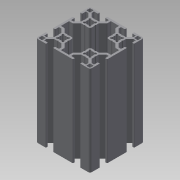
# Autodesk Inventor part: 30-6060
Saved by Autodesk Inventor 2013 (Build 170138000, 138)
## iProperties
Created: 2014-04-23
Part Number: 30-6060
Material: Generic
Document SubType Name: Modeling
Designer: Ross Bowman
Density: 1 g/cm^3
Engineer: Ross Bowman
Catalog Web Link: 8020.net
Vendor: 80/20 Inc.
Company: 80/20 Inc.
Author: Ross Bowman
Keywords: 80/20 , 8020 , T-Slot , Extrusion
Material: 6105-T5 Aluminum
Autodesk Inventor part; units mm, degrees
ref_plane "YZ Plane" through (0, 0, 0) normal (1, 0, 0) x (0, 1, 0)
ref_plane "XZ Plane" through (0, 0, 0) normal (0, 1, 0) x (-1, 0, 0)
ref_plane "XY Plane" through (0, 0, 0) normal (0, 0, 1) x (1, 0, 0)
sketch "Sketch1" plane through (0, 0, 0) normal (0, 0, 1) x (1, 0, 0)
  arc A0 (-28.3189, -24.5) -> (-28.6999, -24.881) centre (-28.3189, -24.881) ccw
  line L0 (-24.88, -24.5) -> (-28.3189, -24.5)
  arc A1 (-24.5, -24.88) -> (-24.88, -24.5) centre (-24.88, -24.88) ccw
  line L1 (-24.5, -28.3189) -> (-24.5, -24.88)
  arc A2 (-24.881, -28.6999) -> (-24.5, -28.3189) centre (-24.881, -28.3189) ccw
  line L2 (-27.6999, -28.6999) -> (-24.881, -28.6999)
  arc A3 (-28.6999, -27.6999) -> (-27.6999, -28.6999) centre (-27.6999, -27.6999) ccw
  line L3 (-28.6999, -24.881) -> (-28.6999, -27.6999)
  arc A4 (24.5, -28.3189) -> (24.881, -28.6999) centre (24.881, -28.3189) ccw
  line L4 (24.5, -24.88) -> (24.5, -28.3189)
  arc A5 (24.88, -24.5) -> (24.5, -24.88) centre (24.88, -24.88) ccw
  line L5 (28.3189, -24.5) -> (24.88, -24.5)
  arc A6 (28.6999, -24.881) -> (28.3189, -24.5) centre (28.3189, -24.881) ccw
  line L6 (28.6999, -27.6999) -> (28.6999, -24.881)
  arc A7 (27.6999, -28.6999) -> (28.6999, -27.6999) centre (27.6999, -27.6999) ccw
  line L7 (24.881, -28.6999) -> (27.6999, -28.6999)
  arc A8 (24.881, 28.6999) -> (24.5, 28.3189) centre (24.881, 28.3189) ccw
  line L8 (27.6999, 28.6999) -> (24.881, 28.6999)
  arc A9 (28.6999, 27.6999) -> (27.6999, 28.6999) centre (27.6999, 27.6999) ccw
  line L9 (28.6999, 24.881) -> (28.6999, 27.6999)
  arc A10 (28.3189, 24.5) -> (28.6999, 24.881) centre (28.3189, 24.881) ccw
  line L10 (24.88, 24.5) -> (28.3189, 24.5)
  arc A11 (24.5, 24.88) -> (24.88, 24.5) centre (24.88, 24.88) ccw
  line L11 (24.5, 28.3189) -> (24.5, 24.88)
  arc A12 (-24.5, 28.3189) -> (-24.881, 28.6999) centre (-24.881, 28.3189) ccw
  line L12 (-24.5, 24.88) -> (-24.5, 28.3189)
  arc A13 (-24.88, 24.5) -> (-24.5, 24.88) centre (-24.88, 24.88) ccw
  line L13 (-28.3189, 24.5) -> (-24.88, 24.5)
  arc A14 (-28.6999, 24.881) -> (-28.3189, 24.5) centre (-28.3189, 24.881) ccw
  line L14 (-28.6999, 27.6999) -> (-28.6999, 24.881)
  arc A15 (-27.6999, 28.6999) -> (-28.6999, 27.6999) centre (-27.6999, 27.6999) ccw
  line L15 (-24.881, 28.6999) -> (-27.6999, 28.6999)
  arc A16 (-16.4942, 11.8018) -> (-13.5057, 11.8018) centre (-15, 15) ccw
  line L16 (-17.4733, 11.02) -> (-16.4942, 11.8018)
  arc A17 (-18.9799, 12.5266) -> (-17.4733, 11.02) centre (-18.1422, 11.8577) ccw
  line L17 (-18.1981, 13.5057) -> (-18.9799, 12.5266)
  arc A18 (-18.1981, 16.4942) -> (-18.1981, 13.5057) centre (-15, 15) ccw
  line L18 (-18.9799, 17.4733) -> (-18.1981, 16.4942)
  arc A19 (-17.4733, 18.9799) -> (-18.9799, 17.4733) centre (-18.1422, 18.1422) ccw
  line L19 (-16.4942, 18.1981) -> (-17.4733, 18.9799)
  arc A20 (-13.5057, 18.1981) -> (-16.4942, 18.1981) centre (-15, 15) ccw
  line L20 (-12.5266, 18.9799) -> (-13.5057, 18.1981)
  arc A21 (-11.02, 17.4733) -> (-12.5266, 18.9799) centre (-11.8577, 18.1422) ccw
  line L21 (-11.8018, 16.4942) -> (-11.02, 17.4733)
  arc A22 (-11.8018, 13.5057) -> (-11.8018, 16.4942) centre (-15, 15) ccw
  line L22 (-11.02, 12.5266) -> (-11.8018, 13.5057)
  arc A23 (-12.5266, 11.02) -> (-11.02, 12.5266) centre (-11.8577, 11.8577) ccw
  line L23 (-13.5057, 11.8018) -> (-12.5266, 11.02)
  arc A24 (13.5057, 11.8018) -> (16.4942, 11.8018) centre (15, 15) ccw
  line L24 (12.5266, 11.02) -> (13.5057, 11.8018)
  arc A25 (11.02, 12.5266) -> (12.5266, 11.02) centre (11.8577, 11.8577) ccw
  line L25 (11.8018, 13.5057) -> (11.02, 12.5266)
  arc A26 (11.8018, 16.4942) -> (11.8018, 13.5057) centre (15, 15) ccw
  line L26 (11.02, 17.4733) -> (11.8018, 16.4942)
  arc A27 (12.5266, 18.9799) -> (11.02, 17.4733) centre (11.8577, 18.1422) ccw
  line L27 (13.5057, 18.1981) -> (12.5266, 18.9799)
  arc A28 (16.4942, 18.1981) -> (13.5057, 18.1981) centre (15, 15) ccw
  line L28 (17.4733, 18.9799) -> (16.4942, 18.1981)
  arc A29 (18.9799, 17.4733) -> (17.4733, 18.9799) centre (18.1422, 18.1422) ccw
  line L29 (18.1981, 16.4942) -> (18.9799, 17.4733)
  arc A30 (18.1981, 13.5057) -> (18.1981, 16.4942) centre (15, 15) ccw
  line L30 (18.9799, 12.5266) -> (18.1981, 13.5057)
  arc A31 (17.4733, 11.02) -> (18.9799, 12.5266) centre (18.1422, 11.8577) ccw
  line L31 (16.4942, 11.8018) -> (17.4733, 11.02)
  arc A32 (-16.4942, -18.1981) -> (-13.5057, -18.1981) centre (-15, -15) ccw
  line L32 (-17.4733, -18.9799) -> (-16.4942, -18.1981)
  arc A33 (-18.9799, -17.4733) -> (-17.4733, -18.9799) centre (-18.1422, -18.1422) ccw
  line L33 (-18.1981, -16.4942) -> (-18.9799, -17.4733)
  arc A34 (-18.1981, -13.5057) -> (-18.1981, -16.4942) centre (-15, -15) ccw
  line L34 (-18.9799, -12.5266) -> (-18.1981, -13.5057)
  arc A35 (-17.4733, -11.02) -> (-18.9799, -12.5266) centre (-18.1422, -11.8577) ccw
  line L35 (-16.4942, -11.8018) -> (-17.4733, -11.02)
  arc A36 (-13.5057, -11.8018) -> (-16.4942, -11.8018) centre (-15, -15) ccw
  line L36 (-12.5266, -11.02) -> (-13.5057, -11.8018)
  arc A37 (-11.02, -12.5266) -> (-12.5266, -11.02) centre (-11.8577, -11.8577) ccw
  line L37 (-11.8018, -13.5057) -> (-11.02, -12.5266)
  arc A38 (-11.8018, -16.4942) -> (-11.8018, -13.5057) centre (-15, -15) ccw
  line L38 (-11.02, -17.4733) -> (-11.8018, -16.4942)
  arc A39 (-12.5266, -18.9799) -> (-11.02, -17.4733) centre (-11.8577, -18.1422) ccw
  line L39 (-13.5057, -18.1981) -> (-12.5266, -18.9799)
  arc A40 (13.5057, -18.1981) -> (16.4942, -18.1981) centre (15, -15) ccw
  line L40 (12.5266, -18.9799) -> (13.5057, -18.1981)
  arc A41 (11.02, -17.4733) -> (12.5266, -18.9799) centre (11.8577, -18.1422) ccw
  line L41 (11.8018, -16.4942) -> (11.02, -17.4733)
  arc A42 (11.8018, -13.5057) -> (11.8018, -16.4942) centre (15, -15) ccw
  line L42 (11.02, -12.5266) -> (11.8018, -13.5057)
  arc A43 (12.5266, -11.02) -> (11.02, -12.5266) centre (11.8577, -11.8577) ccw
  line L43 (13.5057, -11.8018) -> (12.5266, -11.02)
  arc A44 (16.4942, -11.8018) -> (13.5057, -11.8018) centre (15, -15) ccw
  line L44 (17.4733, -11.02) -> (16.4942, -11.8018)
  arc A45 (18.9799, -12.5266) -> (17.4733, -11.02) centre (18.1422, -11.8577) ccw
  line L45 (18.1981, -13.5057) -> (18.9799, -12.5266)
  arc A46 (18.1981, -16.4942) -> (18.1981, -13.5057) centre (15, -15) ccw
  line L46 (18.9799, -17.4733) -> (18.1981, -16.4942)
  arc A47 (17.4733, -18.9799) -> (18.9799, -17.4733) centre (18.1422, -18.1422) ccw
  line L47 (16.4942, -18.1981) -> (17.4733, -18.9799)
  arc A48 (27.7999, 4.05) -> (27.2999, 4.55) centre (27.2999, 4.05) ccw
  line L48 (27.7999, -4.05) -> (27.7999, 4.05)
  arc A49 (27.2999, -4.55) -> (27.7999, -4.05) centre (27.2999, -4.05) ccw
  line L49 (24.2681, -4.55) -> (27.2999, -4.55)
  arc A50 (24.2681, -4.55) -> (23.2075, -4.9893) centre (24.2681, -6.05) ccw
  line L50 (19.178, -9.0188) -> (23.2075, -4.9893)
  arc A51 (18.8244, -9.1653) -> (19.178, -9.0188) centre (18.8244, -8.6653) ccw
  line L51 (15.95, -9.1653) -> (18.8244, -9.1653)
  line L52 (15, -9.6753) -> (15.95, -9.1653)
  line L53 (14.05, -9.1653) -> (15, -9.6753)
  line L54 (11.1653, -9.1653) -> (14.05, -9.1653)
  arc A52 (11.1653, -9.1653) -> (9.1653, -11.1653) centre (11.1653, -11.1653) ccw
  line L55 (9.1653, -14.1125) -> (9.1653, -11.1653)
  line L56 (9.6753, -15.0625) -> (9.1653, -14.1125)
  line L57 (9.1653, -16.0125) -> (9.6753, -15.0625)
  line L58 (9.1653, -18.8244) -> (9.1653, -16.0125)
  arc A53 (9.0188, -19.178) -> (9.1653, -18.8244) centre (8.6653, -18.8244) ccw
  line L59 (4.9893, -23.2075) -> (9.0188, -19.178)
  arc A54 (4.9893, -23.2075) -> (4.55, -24.2681) centre (6.05, -24.2681) ccw
  line L60 (4.55, -27.2999) -> (4.55, -24.2681)
  arc A55 (4.05, -27.7999) -> (4.55, -27.2999) centre (4.05, -27.2999) ccw
  line L61 (-4.05, -27.7999) -> (4.05, -27.7999)
  arc A56 (-4.55, -27.2999) -> (-4.05, -27.7999) centre (-4.05, -27.2999) ccw
  line L62 (-4.55, -24.2681) -> (-4.55, -27.2999)
  arc A57 (-4.55, -24.2681) -> (-4.9893, -23.2075) centre (-6.05, -24.2681) ccw
  line L63 (-9.0188, -19.178) -> (-4.9893, -23.2075)
  arc A58 (-9.1653, -18.8244) -> (-9.0188, -19.178) centre (-8.6653, -18.8244) ccw
  line L64 (-9.1653, -16.0125) -> (-9.1653, -18.8244)
  line L65 (-9.6753, -15.0625) -> (-9.1653, -16.0125)
  line L66 (-9.1653, -14.1125) -> (-9.6753, -15.0625)
  line L67 (-9.1653, -11.1653) -> (-9.1653, -14.1125)
  arc A59 (-9.1653, -11.1653) -> (-11.1653, -9.1653) centre (-11.1653, -11.1653) ccw
  line L68 (-14.05, -9.1653) -> (-11.1653, -9.1653)
  line L69 (-15, -9.6753) -> (-14.05, -9.1653)
  line L70 (-15.95, -9.1653) -> (-15, -9.6753)
  line L71 (-18.8244, -9.1653) -> (-15.95, -9.1653)
  arc A60 (-19.178, -9.0188) -> (-18.8244, -9.1653) centre (-18.8244, -8.6653) ccw
  line L72 (-23.2075, -4.9893) -> (-19.178, -9.0188)
  arc A61 (-23.2075, -4.9893) -> (-24.2681, -4.55) centre (-24.2681, -6.05) ccw
  line L73 (-27.2999, -4.55) -> (-24.2681, -4.55)
  arc A62 (-27.7999, -4.05) -> (-27.2999, -4.55) centre (-27.2999, -4.05) ccw
  line L74 (-27.7999, 4.05) -> (-27.7999, -4.05)
  arc A63 (-27.2999, 4.55) -> (-27.7999, 4.05) centre (-27.2999, 4.05) ccw
  line L75 (-24.2681, 4.55) -> (-27.2999, 4.55)
  arc A64 (-24.2681, 4.55) -> (-23.2075, 4.9893) centre (-24.2681, 6.05) ccw
  line L76 (-19.178, 9.0188) -> (-23.2075, 4.9893)
  arc A65 (-18.8244, 9.1653) -> (-19.178, 9.0188) centre (-18.8244, 8.6653) ccw
  line L77 (-15.95, 9.1653) -> (-18.8244, 9.1653)
  line L78 (-15, 9.6753) -> (-15.95, 9.1653)
  line L79 (-14.05, 9.1653) -> (-15, 9.6753)
  line L80 (-11.1653, 9.1653) -> (-14.05, 9.1653)
  arc A66 (-11.1653, 9.1653) -> (-9.1653, 11.1653) centre (-11.1653, 11.1653) ccw
  line L81 (-9.1653, 13.9875) -> (-9.1653, 11.1653)
  line L82 (-9.6753, 14.9375) -> (-9.1653, 13.9875)
  line L83 (-9.1653, 15.8875) -> (-9.6753, 14.9375)
  line L84 (-9.1653, 18.8244) -> (-9.1653, 15.8875)
  arc A67 (-9.0188, 19.178) -> (-9.1653, 18.8244) centre (-8.6653, 18.8244) ccw
  line L85 (-4.9893, 23.2075) -> (-9.0188, 19.178)
  arc A68 (-4.9893, 23.2075) -> (-4.55, 24.2681) centre (-6.05, 24.2681) ccw
  line L86 (-4.55, 27.2999) -> (-4.55, 24.2681)
  arc A69 (-4.05, 27.7999) -> (-4.55, 27.2999) centre (-4.05, 27.2999) ccw
  line L87 (4.05, 27.7999) -> (-4.05, 27.7999)
  arc A70 (4.55, 27.2999) -> (4.05, 27.7999) centre (4.05, 27.2999) ccw
  line L88 (4.55, 24.2681) -> (4.55, 27.2999)
  arc A71 (4.55, 24.2681) -> (4.9893, 23.2075) centre (6.05, 24.2681) ccw
  line L89 (9.0188, 19.178) -> (4.9893, 23.2075)
  arc A72 (9.1653, 18.8244) -> (9.0188, 19.178) centre (8.6653, 18.8244) ccw
  line L90 (9.1653, 15.8875) -> (9.1653, 18.8244)
  line L91 (9.6753, 14.9375) -> (9.1653, 15.8875)
  line L92 (9.1653, 13.9875) -> (9.6753, 14.9375)
  line L93 (9.1653, 11.1653) -> (9.1653, 13.9875)
  arc A73 (9.1653, 11.1653) -> (11.1653, 9.1653) centre (11.1653, 11.1653) ccw
  line L94 (14.05, 9.1653) -> (11.1653, 9.1653)
  line L95 (15, 9.6753) -> (14.05, 9.1653)
  line L96 (15.95, 9.1653) -> (15, 9.6753)
  line L97 (18.8244, 9.1653) -> (15.95, 9.1653)
  arc A74 (19.178, 9.0188) -> (18.8244, 9.1653) centre (18.8244, 8.6653) ccw
  line L98 (23.2075, 4.9893) -> (19.178, 9.0188)
  arc A75 (23.2075, 4.9893) -> (24.2681, 4.55) centre (24.2681, 6.05) ccw
  line L99 (27.2999, 4.55) -> (24.2681, 4.55)
  arc A76 (-29.9999, -10.5) -> (-29.4999, -11) centre (-29.4999, -10.5) ccw
  line L100 (-29.4999, -11) -> (-28.2425, -11)
  arc A77 (-28.2425, -11) -> (-27.7425, -10.5) centre (-28.2425, -10.5) ccw
  line L101 (-27.7425, -10.5) -> (-27.7425, -7.2674)
  arc A78 (-27.2428, -6.75) -> (-27.7425, -7.2674) centre (-27.2428, -7.25) ccw
  line L102 (-27.2428, -6.75) -> (-25.2602, -6.75)
  arc A79 (-24.9066, -6.8964) -> (-25.2602, -6.75) centre (-25.2602, -7.25) ccw
  line L103 (-24.9066, -6.8964) -> (-20.9811, -10.822)
  arc A80 (-20.8347, -11.1755) -> (-20.9811, -10.822) centre (-21.3347, -11.1755) ccw
  line L104 (-20.8347, -11.1755) -> (-20.8347, -14.1125)
  line L105 (-20.8347, -14.1125) -> (-20.3247, -15.0625)
  line L106 (-20.3247, -15.0625) -> (-20.8347, -16.0125)
  line L107 (-20.8347, -16.0125) -> (-20.8347, -18.8244)
  arc A81 (-20.9811, -19.178) -> (-20.8347, -18.8244) centre (-21.3347, -18.8244) ccw
  line L108 (-20.9811, -19.178) -> (-24.9066, -23.1035)
  arc A82 (-25.2602, -23.25) -> (-24.9066, -23.1035) centre (-25.2602, -22.75) ccw
  line L109 (-25.2602, -23.25) -> (-27.2428, -23.25)
  arc A83 (-27.7425, -22.7325) -> (-27.2428, -23.25) centre (-27.2428, -22.75) ccw
  line L110 (-27.7425, -22.7325) -> (-27.7425, -19.5)
  arc A84 (-27.7425, -19.5) -> (-28.2425, -19) centre (-28.2425, -19.5) ccw
  line L111 (-28.2425, -19) -> (-29.4999, -19)
  arc A85 (-29.4999, -19) -> (-29.9999, -19.5) centre (-29.4999, -19.5) ccw
  line L112 (-29.9999, -19.5) -> (-29.9999, -27.9999)
  arc A86 (-29.9999, -27.9999) -> (-27.9999, -29.9999) centre (-27.9999, -27.9999) ccw
  line L113 (-27.9999, -29.9999) -> (-19.5, -29.9999)
  arc A87 (-19.5, -29.9999) -> (-19, -29.4999) centre (-19.5, -29.4999) ccw
  line L114 (-19, -29.4999) -> (-19, -28.2425)
  arc A88 (-19, -28.2425) -> (-19.5, -27.7425) centre (-19.5, -28.2425) ccw
  line L115 (-19.5, -27.7425) -> (-22.7325, -27.7425)
  arc A89 (-23.25, -27.2428) -> (-22.7325, -27.7425) centre (-22.75, -27.2428) ccw
  line L116 (-23.25, -27.2428) -> (-23.25, -25.2602)
  arc A90 (-23.1035, -24.9066) -> (-23.25, -25.2602) centre (-22.75, -25.2602) ccw
  line L117 (-23.1035, -24.9066) -> (-19.178, -20.9811)
  arc A91 (-18.8244, -20.8347) -> (-19.178, -20.9811) centre (-18.8244, -21.3347) ccw
  line L118 (-18.8244, -20.8347) -> (-15.95, -20.8347)
  line L119 (-15.95, -20.8347) -> (-15, -20.3247)
  line L120 (-15, -20.3247) -> (-14.05, -20.8347)
  line L121 (-14.05, -20.8347) -> (-11.1755, -20.8347)
  arc A92 (-10.822, -20.9811) -> (-11.1755, -20.8347) centre (-11.1755, -21.3347) ccw
  line L122 (-10.822, -20.9811) -> (-6.8964, -24.9066)
  arc A93 (-6.75, -25.2602) -> (-6.8964, -24.9066) centre (-7.25, -25.2602) ccw
  line L123 (-6.75, -25.2602) -> (-6.75, -27.2428)
  arc A94 (-7.2674, -27.7425) -> (-6.75, -27.2428) centre (-7.25, -27.2428) ccw
  line L124 (-7.2674, -27.7425) -> (-10.5, -27.7425)
  arc A95 (-10.5, -27.7425) -> (-11, -28.2425) centre (-10.5, -28.2425) ccw
  line L125 (-11, -28.2425) -> (-11, -29.4999)
  arc A96 (-11, -29.4999) -> (-10.5, -29.9999) centre (-10.5, -29.4999) ccw
  line L126 (-10.5, -29.9999) -> (10.5, -29.9999)
  arc A97 (10.5, -29.9999) -> (11, -29.4999) centre (10.5, -29.4999) ccw
  line L127 (11, -29.4999) -> (11, -28.2425)
  arc A98 (11, -28.2425) -> (10.5, -27.7425) centre (10.5, -28.2425) ccw
  line L128 (10.5, -27.7425) -> (7.2674, -27.7425)
  arc A99 (6.75, -27.2428) -> (7.2674, -27.7425) centre (7.25, -27.2428) ccw
  line L129 (6.75, -27.2428) -> (6.75, -25.2602)
  arc A100 (6.8964, -24.9066) -> (6.75, -25.2602) centre (7.25, -25.2602) ccw
  line L130 (6.8964, -24.9066) -> (10.822, -20.9811)
  arc A101 (11.1755, -20.8347) -> (10.822, -20.9811) centre (11.1755, -21.3347) ccw
  line L131 (11.1755, -20.8347) -> (14.05, -20.8347)
  line L132 (14.05, -20.8347) -> (15, -20.3247)
  line L133 (15, -20.3247) -> (15.95, -20.8347)
  line L134 (15.95, -20.8347) -> (18.8244, -20.8347)
  arc A102 (19.178, -20.9811) -> (18.8244, -20.8347) centre (18.8244, -21.3347) ccw
  line L135 (19.178, -20.9811) -> (23.1035, -24.9066)
  arc A103 (23.25, -25.2602) -> (23.1035, -24.9066) centre (22.75, -25.2602) ccw
  line L136 (23.25, -25.2602) -> (23.25, -27.2428)
  arc A104 (22.7325, -27.7425) -> (23.25, -27.2428) centre (22.75, -27.2428) ccw
  line L137 (22.7325, -27.7425) -> (19.5, -27.7425)
  arc A105 (19.5, -27.7425) -> (19, -28.2425) centre (19.5, -28.2425) ccw
  line L138 (19, -28.2425) -> (19, -29.4999)
  arc A106 (19, -29.4999) -> (19.5, -29.9999) centre (19.5, -29.4999) ccw
  line L139 (19.5, -29.9999) -> (27.9999, -29.9999)
  arc A107 (27.9999, -29.9999) -> (29.9999, -27.9999) centre (27.9999, -27.9999) ccw
  line L140 (29.9999, -27.9999) -> (29.9999, -19.5)
  arc A108 (29.9999, -19.5) -> (29.4999, -19) centre (29.4999, -19.5) ccw
  line L141 (29.4999, -19) -> (28.2425, -19)
  arc A109 (28.2425, -19) -> (27.7425, -19.5) centre (28.2425, -19.5) ccw
  line L142 (27.7425, -19.5) -> (27.7425, -22.7325)
  arc A110 (27.2428, -23.25) -> (27.7425, -22.7325) centre (27.2428, -22.75) ccw
  line L143 (27.2428, -23.25) -> (25.2602, -23.25)
  arc A111 (24.9066, -23.1035) -> (25.2602, -23.25) centre (25.2602, -22.75) ccw
  line L144 (24.9066, -23.1035) -> (20.9811, -19.178)
  arc A112 (20.8347, -18.8244) -> (20.9811, -19.178) centre (21.3347, -18.8244) ccw
  line L145 (20.8347, -18.8244) -> (20.8347, -16.0125)
  line L146 (20.8347, -16.0125) -> (20.3247, -15.0625)
  line L147 (20.3247, -15.0625) -> (20.8347, -14.1125)
  line L148 (20.8347, -14.1125) -> (20.8347, -11.1755)
  arc A113 (20.9811, -10.822) -> (20.8347, -11.1755) centre (21.3347, -11.1755) ccw
  line L149 (20.9811, -10.822) -> (24.9066, -6.8964)
  arc A114 (25.2602, -6.75) -> (24.9066, -6.8964) centre (25.2602, -7.25) ccw
  line L150 (25.2602, -6.75) -> (27.2428, -6.75)
  arc A115 (27.7425, -7.2674) -> (27.2428, -6.75) centre (27.2428, -7.25) ccw
  line L151 (27.7425, -7.2674) -> (27.7425, -10.5)
  arc A116 (27.7425, -10.5) -> (28.2425, -11) centre (28.2425, -10.5) ccw
  line L152 (28.2425, -11) -> (29.4999, -11)
  arc A117 (29.4999, -11) -> (29.9999, -10.5) centre (29.4999, -10.5) ccw
  line L153 (29.9999, -10.5) -> (29.9999, 10.5)
  arc A118 (29.9999, 10.5) -> (29.4999, 11) centre (29.4999, 10.5) ccw
  line L154 (29.4999, 11) -> (28.2425, 11)
  arc A119 (28.2425, 11) -> (27.7425, 10.5) centre (28.2425, 10.5) ccw
  line L155 (27.7425, 10.5) -> (27.7425, 7.2674)
  arc A120 (27.2428, 6.75) -> (27.7425, 7.2674) centre (27.2428, 7.25) ccw
  line L156 (27.2428, 6.75) -> (25.2602, 6.75)
  arc A121 (24.9066, 6.8964) -> (25.2602, 6.75) centre (25.2602, 7.25) ccw
  line L157 (24.9066, 6.8964) -> (20.9811, 10.822)
  arc A122 (20.8347, 11.1755) -> (20.9811, 10.822) centre (21.3347, 11.1755) ccw
  line L158 (20.8347, 11.1755) -> (20.8347, 13.9875)
  line L159 (20.8347, 13.9875) -> (20.3247, 14.9375)
  line L160 (20.3247, 14.9375) -> (20.8347, 15.8875)
  line L161 (20.8347, 15.8875) -> (20.8347, 18.8244)
  arc A123 (20.9811, 19.178) -> (20.8347, 18.8244) centre (21.3347, 18.8244) ccw
  line L162 (20.9811, 19.178) -> (24.9066, 23.1035)
  arc A124 (25.2602, 23.25) -> (24.9066, 23.1035) centre (25.2602, 22.75) ccw
  line L163 (25.2602, 23.25) -> (27.2428, 23.25)
  arc A125 (27.7425, 22.7325) -> (27.2428, 23.25) centre (27.2428, 22.75) ccw
  line L164 (27.7425, 22.7325) -> (27.7425, 19.5)
  arc A126 (27.7425, 19.5) -> (28.2425, 19) centre (28.2425, 19.5) ccw
  line L165 (28.2425, 19) -> (29.4999, 19)
  arc A127 (29.4999, 19) -> (29.9999, 19.5) centre (29.4999, 19.5) ccw
  line L166 (29.9999, 19.5) -> (29.9999, 27.9999)
  arc A128 (29.9999, 27.9999) -> (27.9999, 29.9999) centre (27.9999, 27.9999) ccw
  line L167 (27.9999, 29.9999) -> (19.5, 29.9999)
  arc A129 (19.5, 29.9999) -> (19, 29.4999) centre (19.5, 29.4999) ccw
  line L168 (19, 29.4999) -> (19, 28.2425)
  arc A130 (19, 28.2425) -> (19.5, 27.7425) centre (19.5, 28.2425) ccw
  line L169 (19.5, 27.7425) -> (22.7325, 27.7425)
  arc A131 (23.25, 27.2428) -> (22.7325, 27.7425) centre (22.75, 27.2428) ccw
  line L170 (23.25, 27.2428) -> (23.25, 25.2602)
  arc A132 (23.1035, 24.9066) -> (23.25, 25.2602) centre (22.75, 25.2602) ccw
  line L171 (23.1035, 24.9066) -> (19.178, 20.9811)
  arc A133 (18.8244, 20.8347) -> (19.178, 20.9811) centre (18.8244, 21.3347) ccw
  line L172 (18.8244, 20.8347) -> (15.95, 20.8347)
  line L173 (15.95, 20.8347) -> (15, 20.3247)
  line L174 (15, 20.3247) -> (14.05, 20.8347)
  line L175 (14.05, 20.8347) -> (11.1755, 20.8347)
  arc A134 (10.822, 20.9811) -> (11.1755, 20.8347) centre (11.1755, 21.3347) ccw
  line L176 (10.822, 20.9811) -> (6.8964, 24.9066)
  arc A135 (6.75, 25.2602) -> (6.8964, 24.9066) centre (7.25, 25.2602) ccw
  line L177 (6.75, 25.2602) -> (6.75, 27.2428)
  arc A136 (7.2674, 27.7425) -> (6.75, 27.2428) centre (7.25, 27.2428) ccw
  line L178 (7.2674, 27.7425) -> (10.5, 27.7425)
  arc A137 (10.5, 27.7425) -> (11, 28.2425) centre (10.5, 28.2425) ccw
  line L179 (11, 28.2425) -> (11, 29.4999)
  arc A138 (11, 29.4999) -> (10.5, 29.9999) centre (10.5, 29.4999) ccw
  line L180 (10.5, 29.9999) -> (-10.5, 29.9999)
  arc A139 (-10.5, 29.9999) -> (-11, 29.4999) centre (-10.5, 29.4999) ccw
  line L181 (-11, 29.4999) -> (-11, 28.2425)
  arc A140 (-11, 28.2425) -> (-10.5, 27.7425) centre (-10.5, 28.2425) ccw
  line L182 (-10.5, 27.7425) -> (-7.2674, 27.7425)
  arc A141 (-6.75, 27.2428) -> (-7.2674, 27.7425) centre (-7.25, 27.2428) ccw
  line L183 (-6.75, 27.2428) -> (-6.75, 25.2602)
  arc A142 (-6.8964, 24.9066) -> (-6.75, 25.2602) centre (-7.25, 25.2602) ccw
  line L184 (-6.8964, 24.9066) -> (-10.822, 20.9811)
  arc A143 (-11.1755, 20.8347) -> (-10.822, 20.9811) centre (-11.1755, 21.3347) ccw
  line L185 (-11.1755, 20.8347) -> (-14.05, 20.8347)
  line L186 (-14.05, 20.8347) -> (-15, 20.3247)
  line L187 (-15, 20.3247) -> (-15.95, 20.8347)
  line L188 (-15.95, 20.8347) -> (-18.8244, 20.8347)
  arc A144 (-19.178, 20.9811) -> (-18.8244, 20.8347) centre (-18.8244, 21.3347) ccw
  line L189 (-19.178, 20.9811) -> (-23.1035, 24.9066)
  arc A145 (-23.25, 25.2602) -> (-23.1035, 24.9066) centre (-22.75, 25.2602) ccw
  line L190 (-23.25, 25.2602) -> (-23.25, 27.2428)
  arc A146 (-22.7325, 27.7425) -> (-23.25, 27.2428) centre (-22.75, 27.2428) ccw
  line L191 (-22.7325, 27.7425) -> (-19.5, 27.7425)
  arc A147 (-19.5, 27.7425) -> (-19, 28.2425) centre (-19.5, 28.2425) ccw
  line L192 (-19, 28.2425) -> (-19, 29.4999)
  arc A148 (-19, 29.4999) -> (-19.5, 29.9999) centre (-19.5, 29.4999) ccw
  line L193 (-19.5, 29.9999) -> (-27.9999, 29.9999)
  arc A149 (-27.9999, 29.9999) -> (-29.9999, 27.9999) centre (-27.9999, 27.9999) ccw
  line L194 (-29.9999, 27.9999) -> (-29.9999, 19.5)
  arc A150 (-29.9999, 19.5) -> (-29.4999, 19) centre (-29.4999, 19.5) ccw
  line L195 (-29.4999, 19) -> (-28.2425, 19)
  arc A151 (-28.2425, 19) -> (-27.7425, 19.5) centre (-28.2425, 19.5) ccw
  line L196 (-27.7425, 19.5) -> (-27.7425, 22.7325)
  arc A152 (-27.2428, 23.25) -> (-27.7425, 22.7325) centre (-27.2428, 22.75) ccw
  line L197 (-27.2428, 23.25) -> (-25.2602, 23.25)
  arc A153 (-24.9066, 23.1035) -> (-25.2602, 23.25) centre (-25.2602, 22.75) ccw
  line L198 (-24.9066, 23.1035) -> (-20.9811, 19.178)
  arc A154 (-20.8347, 18.8244) -> (-20.9811, 19.178) centre (-21.3347, 18.8244) ccw
  line L199 (-20.8347, 18.8244) -> (-20.8347, 15.8875)
  line L200 (-20.8347, 15.8875) -> (-20.3247, 14.9375)
  line L201 (-20.3247, 14.9375) -> (-20.8347, 13.9875)
  line L202 (-20.8347, 13.9875) -> (-20.8347, 11.1755)
  arc A155 (-20.9811, 10.822) -> (-20.8347, 11.1755) centre (-21.3347, 11.1755) ccw
  line L203 (-20.9811, 10.822) -> (-24.9066, 6.8964)
  arc A156 (-25.2602, 6.75) -> (-24.9066, 6.8964) centre (-25.2602, 7.25) ccw
  line L204 (-25.2602, 6.75) -> (-27.2428, 6.75)
  arc A157 (-27.7425, 7.2674) -> (-27.2428, 6.75) centre (-27.2428, 7.25) ccw
  line L205 (-27.7425, 7.2674) -> (-27.7425, 10.5)
  arc A158 (-27.7425, 10.5) -> (-28.2425, 11) centre (-28.2425, 10.5) ccw
  line L206 (-28.2425, 11) -> (-29.4999, 11)
  arc A159 (-29.4999, 11) -> (-29.9999, 10.5) centre (-29.4999, 10.5) ccw
  line L207 (-29.9999, 10.5) -> (-29.9999, -10.5)
  point P0 (0, 0)
  constraints: 416 end point, 320 point on circle, 160 centre point
extrude "Extrusion1" add sketch "Sketch1" against normal blind 100
body "Solid1"
